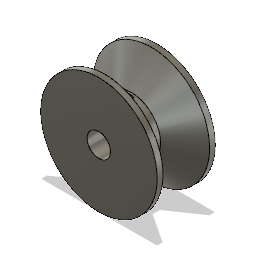
Spindl v1 (Autodesk Fusion 360 design; units mm, degrees)
Autodesk Fusion 360 part; units mm, degrees
sketch "Sketch1" plane through (0, 0, 0) normal (0, 1, 0) x (1, 0, 0)
  line L0 (0, 20) -> (20, 20)
  line L1 (20, 0) -> (0, 0)
  line L2 (0, 20) -> (0, 0)
  line L3 (10, 11.15) -> (10, 8.65)
  line L4 (20, 20) -> (20, 18)
  line L5 (20, 18) -> (10, 11.15)
  line L6 (10, 8.65) -> (20, 2)
  line L7 (20, 2) -> (20, 0)
  dimension "d3" = 20
  dimension "d4" = 20
  dimension "d5" = 10
  dimension "d7" = 2
  dimension "d9" = 2.5
  dimension "d18" = 8.85
  constraint horizontal L0
  constraint coincident L1.end L2.end
  constraint perpendicular L1 L2
  constraint perpendicular L0 L2
  constraint parallel L2 L3
  constraint equal L0 L1
  constraint perpendicular L0 L4
  constraint perpendicular L1 L7
  constraint equal L4 L7
  measures "d3" distance of L0.start L1.end
  measures "d4" distance of L0.start L0.end
  measures "d5" distance of L2 L3
  measures "d7" vertical distance of L1.start L6.end
  measures "d9" distance of L3.start L3.end
  measures "d18" distance of L0 L3.start
revolve "Revolve1" add sketch "Sketch1" angle 360 about axis through (0, 0, 1.75) along (0, 0, 1)
hole "Hole1" at (-0.0164, -0.0454, 0) direction (0, 0, -1) diameter 8 depth 15 tip angle 180
sketch "Sketch2" plane through (0, 0, 0) normal (0, 0, 1) x (1, 0, 0)
sketch "Sketch3" plane through (0, 0, -15) normal (0, 0, 1) x (1, 0, 0)
  circle A0 centre (-0.0164, -0.0454) radius 4
  circle A1 centre (-0.0164, -0.0454) radius 1.5
  dimension "d15" = 3
  constraint concentric A0 A1
  measures "d15" diameter of A1
extrude "Extrude1" cut sketch "Sketch3" against normal blind 17 contours A1
sketch "Sketch4" plane through (0, 0, -20) normal (0, 0, -1) x (-1, 0, 0)
  circle A0 centre (0, 0) radius 20
  circle A1 centre (0, 0) radius 3.5
  circle A2 centre (0.0164, -0.0454) radius 1.5
  dimension "d19" = 7
  constraint coincident A0.centre A1.centre
  measures "d19" diameter of A1
extrude "Extrude2" cut sketch "Sketch4" against normal blind 3 contours A1 | A2
sketch "Sketch5" plane through (0, 0, 0) normal (0, 1, 0) x (1, 0, 0)
  line L0 (-1.7235, 9.4108) -> (1.7051, 9.4108)
  line L1 (1.7051, 9.4108) -> (1.7051, 10.3321)
  line L2 (1.7051, 10.3321) -> (-1.7235, 10.3321)
  line L3 (-1.7235, 10.3321) -> (-1.7235, 9.4108)
  constraint horizontal L0
  constraint vertical L1
  constraint horizontal L2
  constraint vertical L3
extrude "Extrude3" cut sketch "Sketch5" along normal blind 30 and the other way blind 15
